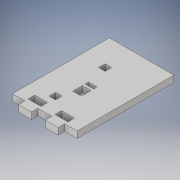
# Autodesk Inventor part: thumper-bumper-sidewall2-v2
Saved by Autodesk Inventor 2017 (Build 210142000, 142)
## iProperties
Created: 2017-02-22
Part Number: thumper-bumper-sidewall2-v2
Material: Generic
Document SubType Name: Modeling
Designer: John
Density: 1 g/cm^3
Appearance: Default
Author: John
Autodesk Inventor part; units mm, degrees
ref_plane "YZ Plane" through (0, 0, 0) normal (1, 0, 0) x (0, 1, 0)
ref_plane "XZ Plane" through (0, 0, 0) normal (0, 1, 0) x (-1, 0, 0)
ref_plane "XY Plane" through (0, 0, 0) normal (0, 0, 1) x (1, 0, 0)
sketch "Sketch1" plane through (0, 0, 0) normal (0, 1, 0) x (-1, 0, 0)
  line L0 (27.5, -0.0615) -> (27.5, 89.9385)
  line L1 (-32.5, 89.9385) -> (-32.5, -0.0615)
  line L2 (-32.5, -0.0615) -> (-2.5, -0.0615)
  line L3 (-2.5, -0.0615) -> (-2.5, 89.9385) construction
  line L4 (-32.5, 44.9385) -> (-2.5, 44.9385) construction
  line L5 (-32.5, 89.9385) -> (27.5, 89.9385)
  line L6 (-21, 89.9385) -> (-9, 89.9385)
  line L7 (-9, 89.9385) -> (-9, 95.9385)
  line L8 (-9, 95.9385) -> (-21, 95.9385)
  line L9 (-21, 95.9385) -> (-21, 89.9385)
  line L10 (16, 89.9385) -> (4, 89.9385)
  line L11 (4, 89.9385) -> (4, 95.9385)
  line L12 (4, 95.9385) -> (16, 95.9385)
  line L13 (16, 95.9385) -> (16, 89.9385)
  line L14 (-2.5, 44.9385) -> (27.5, 44.9385) construction
  line L15 (-2.5, -0.0615) -> (27.5, -0.0615)
  line L16 (-9, 86.9385) -> (-21, 86.9385)
  line L17 (-21, 86.9385) -> (-21, 80.9385)
  line L18 (-21, 80.9385) -> (-9, 80.9385)
  line L19 (-9, 80.9385) -> (-9, 86.9385)
  line L20 (-9, 86.9385) -> (-21, 80.9385) construction
  line L21 (-21, 86.9385) -> (-9, 80.9385) construction
  line L22 (4, 86.9385) -> (16, 86.9385)
  line L23 (16, 86.9385) -> (16, 80.9385)
  line L24 (16, 80.9385) -> (4, 80.9385)
  line L25 (4, 80.9385) -> (4, 86.9385)
  line L26 (4, 86.9385) -> (16, 80.9385) construction
  line L27 (16, 86.9385) -> (4, 80.9385) construction
  point P0 (-15, 83.9385)
  point P1 (10, 83.9385)
  dimension "d0" = 60
  dimension "d1" = 90
  dimension "d18" = 12
  dimension "d19" = 6
  dimension "d20" = 18.5
  dimension "d21" = 12
  dimension "d22" = 6
  dimension "d23" = 3
  constraints: 56 end point, 9 symmetric about line, 7 midpoint, 7 parallel, 5 horizontal, 2 equal length, 2 perpendicular, 1 collinear, 1 point on line, 1 vertical
  measures "d0" distance of L1.start L0.end
  measures "d1" distance of L0.end L0.start
  measures "d18" distance of L8.end L7.end
  measures "d19" distance of L7.end L6.end
  measures "d20" distance between parallel lines of L3 L9
  measures "d21" distance of L18.end L17.end
  measures "d22" distance of L17.end L16.end
  measures "d23" distance between parallel lines of L5 L16
extrude "Extrusion1" add sketch "Sketch1" along normal blind 6
sketch "Sketch3" plane through (0, 0, 0) normal (0, 1, 0) x (-1, 0, 0)
  line L0 (4, 89.9385) -> (-9, 89.9385) construction
  line L1 (-2.5, 89.9385) -> (-2.5, -0.0615) construction
  line L2 (-32.5, -0.0615) -> (27.5, -0.0615) construction
  line L3 (8.5, 74.9385) -> (2.5, 74.9385)
  line L4 (2.5, 74.9385) -> (2.5, 68.9385)
  line L5 (2.5, 68.9385) -> (8.5, 68.9385)
  line L6 (8.5, 68.9385) -> (8.5, 74.9385)
  line L7 (8.5, 28.9385) -> (2.5, 28.9385)
  line L8 (2.5, 28.9385) -> (2.5, 22.9385)
  line L9 (2.5, 22.9385) -> (8.5, 22.9385)
  line L10 (8.5, 22.9385) -> (8.5, 28.9385)
  line L11 (1.5, 59.9385) -> (-6.5, 59.9385)
  line L12 (-6.5, 59.9385) -> (-6.5, 50.9385)
  line L13 (-6.5, 50.9385) -> (1.5, 50.9385)
  line L14 (1.5, 50.9385) -> (1.5, 59.9385)
  line L15 (1.5, 48.4385) -> (-6.5, 48.4385)
  line L16 (-6.5, 48.4385) -> (-6.5, 45.4385)
  line L17 (-6.5, 45.4385) -> (1.5, 45.4385)
  line L18 (1.5, 45.4385) -> (1.5, 48.4385)
  point P0 (0, 0)
  dimension "d37" = 6
  dimension "d38" = 6
  dimension "d39" = 6
  dimension "d43" = 15
  dimension "d44" = 40
  dimension "d45" = 5
  dimension "d46" = 8
  dimension "d47" = 9
  dimension "d48" = 30
  dimension "d49" = 1
  dimension "d50" = 3
  dimension "d51" = 2.5
  constraints: 34 end point, 8 parallel, 4 horizontal, 4 perpendicular, 2 collinear, 2 midpoint
  measures "d37" distance of L5.end L4.end
  measures "d38" distance of L4.end L3.end
  measures "d39" distance of L8.end L7.end
  measures "d43" distance between parallel lines of L0 L3
  measures "d44" distance between parallel lines of L7 L5
  measures "d45" distance between parallel lines of L1 L4
  measures "d46" distance of L13.end L12.end
  measures "d47" distance of L12.end L11.end
  measures "d48" distance between parallel lines of L0 L11
  measures "d49" distance between parallel lines of L4 L14
  measures "d50" distance of L16.end L15.end
  measures "d51" distance between parallel lines of L13 L15
extrude "Extrusion3" cut sketch "Sketch3" along normal through all
body "Solid1"
